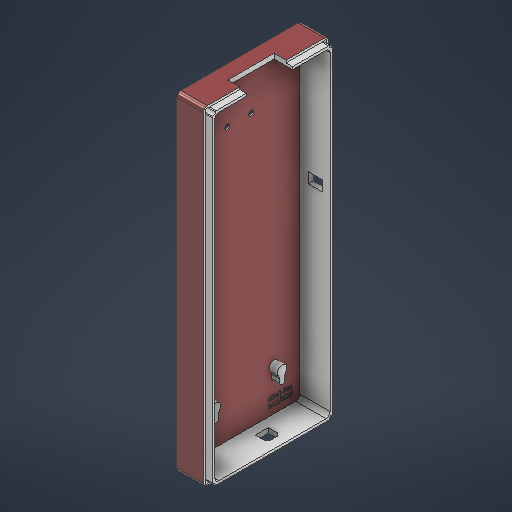
# Autodesk Inventor part: cDAQ_Bottom_Box3
Saved by Autodesk Inventor 2027 (Build 310192000, 192)
## iProperties
Created: 2026-05-08
Part Number: cDAQ_Bottom_Box3
Material: Generic
Document SubType Name: Modeling
Designer: giese
Density: 1 g/cm^3
Appearance: Default
Author: giese
Autodesk Inventor part; units mm, degrees
ref_plane "YZ Plane" through (0, 0, 0) normal (1, 0, 0) x (0, 1, 0)
ref_plane "XZ Plane" through (0, 0, 0) normal (0, 1, 0) x (-1, 0, 0)
ref_plane "XY Plane" through (0, 0, 0) normal (0, 0, 1) x (1, 0, 0)
sketch "Sketch1" plane through (0, 0, 0) normal (1, 0, 0) x (0, 1, 0)
  line L0 (37.5698, 48.0867) -> (-215.7952, 48.0867)
  line L1 (-215.7952, 48.0867) -> (-215.7952, -48.4333)
  line L2 (-215.7952, -48.4333) -> (37.5698, -48.4333)
  line L3 (37.5698, -48.4333) -> (37.5698, 48.0867)
  point P0 (0, 0)
  dimension "d0" = 96.52
  dimension "d1" = 253.365
  constraints: 8 end point, 2 parallel, 1 horizontal, 1 perpendicular
  measures "d0" distance of L2.end L0.start
  measures "d1" distance of L1.end L2.end
extrude "Extrusion1" add sketch "Sketch1" along normal blind 20.32
sketch "Sketch2" plane through (20.32, 0, 0) normal (1, 0, 0) x (0, 0, -1)
  line L0 (44.6233, 33.7598) -> (-44.2767, 33.7598)
  line L1 (-44.2767, 33.7598) -> (-44.2767, -211.9852)
  line L2 (-44.2767, -211.9852) -> (44.6233, -211.9852)
  line L3 (44.6233, -211.9852) -> (44.6233, 33.7598)
  line L4 (48.4333, 37.5698) -> (-48.0867, 37.5698) projected
  line L5 (-48.0867, 37.5698) -> (-48.0867, -215.7952) projected
  point P0 (0, 0)
  dimension "d4" = 245.745
  dimension "d5" = 88.9
  dimension "d8" = 3.81
  dimension "d21" = 3.81
  constraints: 8 end point, 2 parallel, 1 horizontal, 1 perpendicular
  measures "d4" distance of L2.end L0.start
  measures "d5" distance of L0.start L0.end
  measures "d8" distance between parallel lines of L0 L4
  measures "d21" distance between parallel lines of L5 L1
extrude "Extrusion2" cut sketch "Sketch2" against normal blind 18.415
sketch "Sketch3" plane through (0, 0, 0) normal (-1, 0, 0) x (0, 0, 1)
  circle A0 centre (-7.1989, -2.6638) radius 2
  circle A1 centre (11.2999, -2.6638) radius 2
  circle A2 centre (29.7987, -2.6638) radius 2
  line L0 (-48.4333, -215.7952) -> (-48.4333, 37.5698) projected
  line L1 (-48.4333, 37.5698) -> (48.0867, 37.5698) projected
  line L2 (48.0867, 37.5698) -> (48.0867, -215.7952) projected
  line L3 (44.2767, 33.7598) -> (-44.6233, 33.7598) projected
  point P0 (0, 0)
  point P1 (-0.896, -23.7433)
  point P2 (-45.1848, 27.0137)
  dimension "d9" = 18.4988
  dimension "d10" = 4
  dimension "d11" = 4
  dimension "d12" = 18.4988
  dimension "d13" = 36.9976
  dimension "d18" = 18.288
  dimension "d22" = 4
  dimension "d58" = 40.2336
  constraints: 3 centre point
  measures "d9" distance of A0.centre A1.centre
  measures "d10" diameter of A1
  measures "d11" diameter of A2
  measures "d12" distance of A1.centre A2.centre
  measures "d13" distance of A0.centre A2.centre
  measures "d18" distance from line of L2 A2.centre
  measures "d22" diameter of A0
  measures "d58" distance from line of L1 A2.centre
extrude "Extrusion3" cut sketch "Sketch3" against normal blind 3.81
sketch "Sketch5" plane through (0, -215.7952, -48.4333) normal (0, 0, -1) x (-1, 0, 0)
  line L0 (-19.2532, 150.6728) -> (-8.5598, 150.6728)
  line L1 (-8.5598, 150.6728) -> (-8.5598, 158.6728)
  line L2 (-8.5598, 158.6728) -> (-19.2532, 158.6728)
  line L3 (-19.2532, 158.6728) -> (-19.2532, 150.6728)
  line L4 (0, 253.365) -> (-20.32, 253.365) projected
  line L5 (0, 0) -> (0, 253.365) projected
  point P0 (0, 215.7952)
  point P1 (-13.9065, 158.6728)
  point P2 (-13.9065, 150.6728)
  dimension "d28" = 10.6934
  dimension "d30" = 8
  dimension "d31" = 8.5598
  dimension "d34" = 102.6922
  constraints: 8 end point, 2 midpoint, 2 parallel, 1 horizontal, 1 perpendicular
  measures "d28" distance between parallel lines of L1 L3
  measures "d30" distance of point (-13.907, 158.673) point (-13.907, 150.673)
  measures "d31" distance between parallel lines of L5 L1
  measures "d34" distance between parallel lines of L4 L0
extrude "Extrusion4" cut sketch "Sketch5" against normal blind 24.13
sketch "Sketch6" plane through (0, -215.7952, -48.4333) normal (0, -1, 0) x (1, 0, 0)
  line L0 (16, 45.1284) -> (9, 45.1284)
  line L1 (9, 45.1284) -> (9, 35.1284)
  line L2 (9, 35.1284) -> (16, 35.1284)
  line L3 (0, 96.52) -> (0, 0) projected
  line L4 (18.24, 43.1283) -> (18.24, 37.1284)
  line L5 (16, 45.1284) -> (18.24, 43.1283)
  line L6 (18.24, 37.1284) -> (16, 35.1284)
  line L7 (0, 0) -> (20.32, 0) projected
  point P0 (0, 48.4333)
  point P1 (12.5, 45.1284)
  point P2 (12.5, 35.1284)
  dimension "d35" = 10
  dimension "d39" = 6
  dimension "d48" = 45.1284
  dimension "d49" = 18.24
  constraints: 12 end point, 2 midpoint, 1 horizontal, 1 parallel, 1 perpendicular, 1 vertical
  measures "d35" distance of point (12.5, 45.128) point (12.5, 35.128)
  measures "d39" distance of L4.start L4.end
  measures "d48" distance between parallel lines of L7 L0
  measures "d49" distance between parallel lines of L3 L4
extrude "Extrusion5" cut sketch "Sketch6" against normal blind 3.81
sketch "Sketch7" plane through (0, 37.5698, 48.0867) normal (0, 1, 0) x (1, 0, 0)
  line L0 (26.1366, 63.754) -> (11.1252, 63.754)
  line L1 (11.1252, 63.754) -> (11.1252, 28.194)
  line L2 (11.1252, 28.194) -> (26.1366, 28.194)
  line L3 (26.1366, 28.194) -> (26.1366, 63.754)
  line L4 (0, 0) -> (20.32, 0) projected
  line L5 (0, 96.52) -> (0, 0) projected
  line L6 (20.32, 96.52) -> (20.32, 0) projected
  point P0 (0, 48.0867)
  dimension "d51" = 35.56
  dimension "d52" = 28.194
  dimension "d55" = 11.1252
  dimension "d56" = 15.0114
  dimension "d57" = 5.8166
  constraints: 8 end point, 2 parallel, 1 horizontal, 1 perpendicular
  measures "d51" distance of L2.end L0.start
  measures "d52" distance between parallel lines of L4 L2
  measures "d55" distance between parallel lines of L5 L1
  measures "d56" distance between parallel lines of L3 L1
  measures "d57" distance between parallel lines of L6 L3
extrude "Extrusion6" cut sketch "Sketch7" against normal blind 7.62
fillet "Fillet1" radius 3.175 4 edges at (10.16, 37.5698, -48.4333) (10.16, 37.5698, 48.0867) (10.16, -215.7952, -48.4333) (10.16, -215.7952, 48.0867)
sketch "Sketch8" plane through (0, 0, 0) normal (-1, 0, 0) x (0, 0, 1)
  line L0 (-8.9705, -6.1944) -> (-5.4399, -6.1944)
  line L1 (-8.9705, 0.8668) -> (-5.4399, 0.8668)
  line L2 (-8.9705, -6.1944) -> (-11.0089, -2.6638)
  line L3 (-8.9705, 0.8668) -> (-11.0089, -2.6638)
  line L4 (-5.4399, -6.1944) -> (-3.4016, -2.6638)
  line L5 (-5.4399, 0.8668) -> (-3.4016, -2.6638)
  circle A0 centre (-7.1989, -2.6638) radius 2 projected
  line L6 (9.5283, -6.1944) -> (13.0589, -6.1944)
  line L7 (9.5283, 0.8668) -> (13.0589, 0.8668)
  line L8 (9.5283, -6.1944) -> (7.4899, -2.6638)
  line L9 (9.5283, 0.8668) -> (7.4899, -2.6638)
  line L10 (13.0589, -6.1944) -> (15.0973, -2.6638)
  line L11 (13.0589, 0.8668) -> (15.0973, -2.6638)
  circle A1 centre (11.2999, -2.6638) radius 2 projected
  line L12 (28.0271, -6.1944) -> (25.9887, -2.6638)
  line L13 (28.0271, 0.8668) -> (25.9887, -2.6638)
  line L14 (28.0271, -6.1944) -> (31.5577, -6.1944)
  line L15 (28.0271, 0.8668) -> (31.5577, 0.8668)
  line L16 (31.5577, -6.1944) -> (33.5961, -2.6638)
  line L17 (31.5577, 0.8668) -> (33.5961, -2.6638)
  circle A2 centre (29.7987, -2.6638) radius 2 projected
  point P0 (-7.2052, -6.1944)
  point P1 (11.2936, -6.1944)
  point P2 (29.7924, -6.1944)
  point P3 (-11.0089, -2.6638)
  point P4 (-3.4016, -2.6638)
  point P5 (15.0973, -2.6638)
  point P6 (7.4899, -2.6638)
  point P7 (33.5961, -2.6638)
  point P8 (25.9887, -2.6638)
  dimension "d60" = 7.0612
  dimension "d61" = 120
  dimension "d62" = 120
  dimension "d63" = 120
  dimension "d64" = 120
  dimension "d65" = 3.5306
  dimension "d66" = 3.5306
  dimension "d67" = 3.5306
  dimension "d68" = 3.5306
  dimension "d69" = 3.5306
  dimension "d70" = 3.5306
  dimension "d71" = 0
  dimension "d72" = 7.6074
  dimension "d73" = 3.81
  dimension "d74" = 0
  dimension "d75" = 7.0612
  dimension "d76" = 120
  dimension "d77" = 120
  dimension "d78" = 120
  dimension "d79" = 120
  dimension "d80" = 3.5306
  dimension "d81" = 3.5306
  dimension "d82" = 3.5306
  dimension "d83" = 3.5306
  dimension "d84" = 3.5306
  dimension "d85" = 3.5306
  dimension "d86" = 0
  dimension "d87" = 7.6074
  dimension "d91" = 0
  dimension "d92" = 3.81
  dimension "d93" = 7.0612
  dimension "d94" = 120
  dimension "d95" = 120
  dimension "d96" = 120
  dimension "d97" = 120
  dimension "d98" = 3.5306
  dimension "d99" = 3.5306
  dimension "d100" = 3.5306
  dimension "d101" = 3.5306
  dimension "d102" = 3.5306
  dimension "d103" = 3.5306
  dimension "d104" = 0
  dimension "d105" = 7.6074
  dimension "d108" = 0
  dimension "d109" = 3.81
  constraints: 36 end point, 6 horizontal, 3 midpoint
  measures "d60" distance from line of point (-7.205, -6.194) L1
  measures "d61" angle of L0 L2
  measures "d62" angle of L1 L3
  measures "d63" angle of L4 L0
  measures "d64" angle of L5 L1
  measures "d65" distance of L0.start L0.end
  measures "d66" distance of L1.start L1.end
  measures "d67" vertical distance of L1.start L3.end
  measures "d68" vertical distance of L0.start L2.end
  measures "d69" vertical distance of L1.end L5.end
  measures "d70" vertical distance of L0.end L4.end
  measures "d71" horizontal distance of L0.start L1.start
  measures "d72" distance of L4.end L2.end
  measures "d73" distance of A0.centre L2.end
  measures "d74" vertical distance of A0.centre L4.end
  measures "d75" distance from line of point (11.294, -6.194) L7
  measures "d76" angle of L6 L8
  measures "d77" angle of L7 L9
  measures "d78" angle of L10 L6
  measures "d79" angle of L11 L7
  measures "d80" distance of L8.start L6.end
  measures "d81" distance of L9.start L7.end
  measures "d82" vertical distance of L9.start L9.end
  measures "d83" vertical distance of L8.start L8.end
  measures "d84" vertical distance of L7.end L11.end
  measures "d85" vertical distance of L6.end L10.end
  measures "d86" horizontal distance of L8.start L9.start
  measures "d87" distance of L10.end L8.end
  measures "d91" vertical distance of A1.centre L8.end
  measures "d92" distance of A1.centre L8.end
  measures "d93" distance from line of point (29.792, -6.194) L15
  measures "d94" angle of L14 L12
  measures "d95" angle of L15 L13
  measures "d96" angle of L16 L14
  measures "d97" angle of L17 L15
  measures "d98" distance of L12.start L16.start
  measures "d99" distance of L15.start L15.end
  measures "d100" vertical distance of L15.start L13.end
  measures "d101" vertical distance of L12.start L12.end
  measures "d102" vertical distance of L15.end L17.end
  measures "d103" vertical distance of L16.start L16.end
  measures "d104" horizontal distance of L12.start L15.start
  measures "d105" distance of L16.end L12.end
  measures "d108" vertical distance of A2.centre L12.end
  measures "d109" distance of A2.centre L12.end
extrude "Extrusion7" cut sketch "Sketch8" against normal blind 0.9525 contours L2 L3 L1 L5 L4 L0 | A0 | L8 L9 L7 L11 L10 L6 | A1 | L12 L13 L15 L17 L16 L14 | A2
sketch "Sketch9" plane through (1.905, 0, 0) normal (1, 0, 0) x (0, 0, -1)
  arc A0 (27.3489, -182.3284) -> (21.8927, -182.3284) centre (24.6208, -179.8542) ccw
  line L0 (45.2583, 37.5698) -> (15.6673, 37.5698) projected
  line L1 (44.6233, 33.7598) -> (44.6233, -211.9852) projected
  arc A1 (22.7158, -187.4742) -> (26.5258, -187.4742) centre (24.6208, -187.4742) ccw
  line L2 (26.5258, -187.4742) -> (26.5258, -184.4614)
  line L3 (22.7158, -187.4742) -> (22.7158, -184.4614)
  arc A2 (27.3489, -182.3284) -> (26.5258, -184.4614) centre (29.7008, -184.4614) ccw
  arc A3 (22.7158, -184.4614) -> (21.8927, -182.3284) centre (19.5408, -184.4614) ccw
  arc A4 (-23.4511, -182.3284) -> (-28.9073, -182.3285) centre (-26.1792, -179.8542) ccw
  arc A5 (-28.0842, -187.4606) -> (-24.2742, -187.4742) centre (-26.1792, -187.4742) ccw
  line L4 (-24.2742, -187.4742) -> (-24.2742, -184.4614)
  line L5 (-28.0842, -187.4606) -> (-28.0842, -184.4614)
  arc A6 (-23.4511, -182.3284) -> (-24.2742, -184.4614) centre (-21.0992, -184.4614) ccw
  arc A7 (-28.0842, -184.4614) -> (-28.9073, -182.3285) centre (-31.2592, -184.4614) ccw
  line L6 (-19.8927, 37.5698) -> (-44.9117, 37.5698) projected
  line L7 (-44.2767, -211.9852) -> (-44.2767, 33.7598) projected
  point P0 (0, 0)
  point P1 (26.5258, -183.0063)
  point P2 (22.7158, -183.0063)
  point P3 (-24.2742, -183.0063)
  point P4 (-28.0842, -183.0063)
  dimension "d112" = 217.424
  dimension "d114" = 7.366
  dimension "d116" = 3.81
  dimension "d117" = 225.044
  dimension "d118" = 3.175
  dimension "d119" = 7.366
  dimension "d120" = 3.81
  dimension "d121" = 3.175
  dimension "d122" = 217.424
  dimension "d123" = 225.044
  dimension "d125" = 0
  dimension "d128" = 50.8
  dimension "d129" = 20.0025
  dimension "d130" = 0
  constraints: 20 point on circle, 8 centre point, 8 end point, 8 tangent, 4 point on line, 2 equal radius, 2 parallel, 2 vertical
  measures "d112" distance from line of L0 A0.centre
  measures "d114" diameter of A0
  measures "d116" diameter of A1
  measures "d117" distance from line of L0 A1.centre
  measures "d118" radius of A2
  measures "d119" diameter of A4
  measures "d120" diameter of A5
  measures "d121" radius of A6
  measures "d122" distance from line of A4.centre L6
  measures "d123" distance from line of L6 A5.centre
  measures "d125" horizontal distance of A5.centre A4.centre
  measures "d128" distance of A5.centre A1.centre
  measures "d129" distance from line of L1 A0.centre
  measures "d130" horizontal distance of A0.centre A1.centre
extrude "Extrusion8" add sketch "Sketch9" along normal blind 6.4008
sketch "Sketch10" plane through (20.32, 0, 0) normal (1, 0, 0) x (0, 0, -1)
  line L0 (44.6233, -211.9852) -> (-44.2767, -211.9852) projected
  line L1 (-44.2767, -211.9852) -> (-44.2767, 33.7598) projected
  line L2 (-44.2767, -211.9852) -> (-44.2767, -209.6992)
  line L3 (-46.2767, -211.4452) -> (-46.2767, -213.9852)
  line L4 (-46.2767, -213.9852) -> (-41.9907, -213.9852)
  line L5 (-44.2767, -211.9852) -> (-41.9907, -211.9852)
  line L6 (44.6233, -211.9852) -> (42.3373, -211.9852)
  line L7 (42.3373, -213.9852) -> (46.6233, -213.9852)
  line L8 (46.6233, -213.9852) -> (46.6233, -209.6992)
  line L9 (44.6233, 33.7598) -> (44.6233, -211.9852) projected
  line L10 (-44.2767, -209.6992) -> (-44.2767, 33.7598)
  line L11 (-44.2767, 33.7598) -> (44.6233, 33.7598) projected
  line L12 (-41.9907, 35.7598) -> (-46.2767, 35.7598)
  line L13 (-46.2767, 35.7598) -> (-46.2767, 29.7278)
  line L14 (42.3373, 33.7598) -> (44.6233, 33.7598)
  line L15 (46.6233, 31.4738) -> (46.6233, 35.7598)
  line L16 (46.6233, 35.7598) -> (42.3373, 35.7598)
  line L17 (-41.9907, -213.9852) -> (42.3373, -213.9852)
  line L18 (42.3373, -211.9852) -> (-41.9907, -211.9852)
  line L19 (46.6233, -209.6992) -> (46.6233, 31.4738)
  line L20 (44.6233, 31.4738) -> (44.6233, -209.6992)
  line L21 (42.3373, 33.7598) -> (-41.9907, 33.7598)
  line L22 (-41.9907, 35.7598) -> (42.3373, 35.7598)
  line L23 (-44.2767, -209.6992) -> (-44.2767, -209.6992)
  line L24 (-46.2767, 29.7278) -> (-46.2767, -211.4452)
  point P0 (-41.9907, -213.8582)
  point P1 (-44.4037, -209.6992)
  point P2 (-46.2767, 32.7438)
  point P3 (44.6233, 31.4738)
  point P4 (42.3373, 35.7598)
  dimension "d139" = 2
  dimension "d142" = 2
  dimension "d143" = 2
  dimension "d146" = 2
  dimension "d147" = 2
  dimension "d150" = 2
  dimension "d151" = 2
  dimension "d159" = 2
  constraints: 42 end point, 7 point on line, 4 perpendicular, 3 horizontal, 3 parallel, 2 vertical, 1 collinear, 1 midpoint
  measures "d139" distance between parallel lines of L0 L4
  measures "d142" distance between parallel lines of L6 L7
  measures "d143" distance between parallel lines of L9 L8
  measures "d146" distance from line of point (-46.277, 32.744) L1
  measures "d147" distance between parallel lines of L11 L12
  measures "d150" distance between parallel lines of L11 L16
  measures "d151" distance between parallel lines of L9 L15
  measures "d159" distance from line of L1 L3.start
extrude "Extrusion9" add sketch "Sketch10" along normal blind 5
sketch "Sketch11" plane through (20.32, 35.7598, 19.8927) normal (0, 1, 0) x (1, 0, 0)
  line L0 (0, 35.56) -> (-9.1948, 35.56) projected
  line L1 (5, 66.516) -> (5, -26.384) projected
  line L2 (0, 35.56) -> (5, 35.56)
  line L3 (5, 35.56) -> (5, 0)
  line L4 (5, 0) -> (0, 0)
  line L5 (0, 0) -> (0, 35.56)
  point P0 (-20.32, 19.8927)
  point P1 (2.5, 0)
  point P2 (2.5, 35.56)
  point P3 (5, 35.56)
  dimension "d156" = 35.56
  constraints: 8 end point, 2 midpoint, 2 parallel, 1 horizontal, 1 perpendicular, 1 point on line
  measures "d156" distance of point (2.5, 0) point (2.5, 35.56)
extrude "Extrusion10" cut sketch "Sketch11" against normal blind 9.8425
fillet "Fillet2" radius 3.175 8 edges at (22.82, 35.7598, -46.6233) (22.82, 35.7598, 46.2767) (22.82, -213.9852, 46.2767) (22.82, -213.9852, -46.6233) (13.6125, 33.7598, -44.6233) (13.6125, 33.7598, 44.2767) (13.6125, -211.9852, 44.2767) (13.6125, -211.9852, -44.6233)
sketch "Sketch13" plane through (25.32, 0, 0) normal (1, 0, 0) x (0, 0, -1)
  arc A0 (46.6233, 32.5848) -> (43.4483, 35.7598) centre (43.4483, 32.5848) ccw projected
  arc A1 (-43.1017, 35.7598) -> (-46.2767, 32.5848) centre (-43.1017, 32.5848) ccw projected
  circle A2 centre (-45.3344, 34.8421) radius 1.5
  arc A3 (43.4483, -213.9852) -> (46.6233, -210.8102) centre (43.4483, -210.8102) ccw projected
  circle A4 centre (45.681, -213.0676) radius 1.5
  arc A5 (-46.2767, -210.8102) -> (-43.1017, -213.9852) centre (-43.1017, -210.8102) ccw projected
  circle A6 centre (-45.3344, -213.0676) radius 1.5
  circle A7 centre (45.681, 34.8421) radius 1.5
  line L0 (-19.8927, 37.5698) -> (-44.9117, 37.5698) projected
  line L1 (-48.0867, 34.3948) -> (-48.0867, -212.6202) projected
  point P0 (0, 0)
  point P1 (-45.3468, 34.8298)
  dimension "d166" = 3
  dimension "d167" = 3
  dimension "d168" = 3
  dimension "d169" = 3
  dimension "d170" = 2.7399
  dimension "d171" = 2.7523
  constraints: 5 point on circle, 4 centre point
  measures "d166" diameter of A6
  measures "d167" diameter of A4
  measures "d168" diameter of A2
  measures "d169" diameter of A7
  measures "d170" distance from line of L0 point (-45.347, 34.83)
  measures "d171" distance from line of L1 A2.centre
extrude "Extrusion11" cut sketch "Sketch13" against normal blind 25.4
sketch "Sketch14" plane through (1.905, 0, 0) normal (1, 0, 0) x (0, 0, -1)
  line L0 (20.2548, -198.8409) -> (39.4715, -198.8409) construction
  line L1 (39.4715, -198.8409) -> (39.4715, -207.6335) construction
  line L2 (39.4715, -207.6335) -> (20.2548, -207.6335) construction
  line L3 (20.2548, -207.6335) -> (20.2548, -198.8409) construction
  spline S0 degree 2 poles (21.4428, -202.005) (21.2057, -202.005) (20.813, -201.8592) (20.6722, -201.711) knots 0 0 0 1 2 2 2
  spline S1 degree 2 poles (20.6722, -201.711) (20.5314, -201.5653) (20.3758, -201.1158) (20.3758, -200.8144) knots 0 0 0 1 2 2 2
  spline S2 degree 2 poles (20.3758, -200.8144) (20.3758, -200.5131) (20.5363, -200.0734) (20.6722, -199.9252) knots 0 0 0 1 2 2 2
  spline S3 degree 2 poles (20.6722, -199.9252) (20.808, -199.7745) (21.2107, -199.614) (21.4428, -199.614) knots 0 0 0 1 2 2 2
  spline S4 degree 2 poles (21.4428, -199.614) (21.6306, -199.614) (21.9813, -199.7202) (22.1172, -199.7894) knots 0 0 0 1 2 2 2
  line L4 (22.1172, -199.7894) -> (22.1172, -200.2216)
  line L5 (22.1172, -200.2216) -> (22.0949, -200.2216)
  spline S5 degree 2 poles (22.0949, -200.2216) (22.0529, -200.187) (21.9245, -200.0981) (21.8331, -200.0512) knots 0 0 0 1 2 2 2
  spline S6 degree 2 poles (21.8331, -200.0512) (21.7516, -200.0117) (21.5342, -199.9499) (21.4354, -199.9499) knots 0 0 0 1 2 2 2
  spline S7 degree 2 poles (21.4354, -199.9499) (21.1366, -199.9499) (20.7735, -200.4019) (20.7735, -200.8144) knots 0 0 0 1 2 2 2
  spline S8 degree 2 poles (20.7735, -200.8144) (20.7735, -201.217) (21.1242, -201.669) (21.4354, -201.669) knots 0 0 0 1 2 2 2
  spline S9 degree 2 poles (21.4354, -201.669) (21.6231, -201.669) (21.964, -201.5134) (22.0949, -201.3924) knots 0 0 0 1 2 2 2
  line L6 (22.0949, -201.3924) -> (22.1172, -201.3924)
  line L7 (22.1172, -201.3924) -> (22.1172, -201.8247)
  spline S10 degree 2 poles (22.1172, -201.8247) (22.0603, -201.8518) (21.8874, -201.9284) (21.8183, -201.9457) knots 0 0 0 1 2 2 2
  spline S11 degree 2 poles (21.8183, -201.9457) (21.7195, -201.9753) (21.5639, -202.005) (21.4428, -202.005) knots 0 0 0 1 2 2 2
  spline S12 degree 2 poles (24.9009, -200.4316) (24.9009, -200.849) (24.5625, -201.5208) (24.2784, -201.7086) knots 0 0 0 1 2 2 2
  spline S13 degree 2 poles (24.2784, -201.7086) (24.0462, -201.8543) (23.5695, -201.9531) (23.199, -201.9531) knots 0 0 0 1 2 2 2
  line L8 (23.199, -201.9531) -> (22.4975, -201.9531)
  line L9 (22.4975, -201.9531) -> (22.4975, -198.9051)
  line L10 (22.4975, -198.9051) -> (23.1916, -198.9051)
  spline S14 degree 2 poles (23.1916, -198.9051) (23.6214, -198.9051) (24.1105, -199.0335) (24.2834, -199.1472) knots 0 0 0 1 2 2 2
  spline S15 degree 2 poles (24.2834, -199.1472) (24.5773, -199.3423) (24.9009, -199.987) (24.9009, -200.4316) knots 0 0 0 1 2 2 2
  spline S16 degree 2 poles (24.4785, -200.4266) (24.4785, -200.0759) (24.2463, -199.5794) (24.0166, -199.4386) knots 0 0 0 1 2 2 2
  spline S17 degree 2 poles (24.0166, -199.4386) (23.8536, -199.3423) (23.4855, -199.2558) (23.2114, -199.2558) knots 0 0 0 1 2 2 2
  line L11 (23.2114, -199.2558) -> (22.9026, -199.2558)
  line L12 (22.9026, -199.2558) -> (22.9026, -201.6024)
  line L13 (22.9026, -201.6024) -> (23.2114, -201.6024)
  spline S18 degree 2 poles (23.2114, -201.6024) (23.4806, -201.6024) (23.8882, -201.5159) (24.0536, -201.3998) knots 0 0 0 1 2 2 2
  spline S19 degree 2 poles (24.0536, -201.3998) (24.2661, -201.2566) (24.4785, -200.7823) (24.4785, -200.4266) knots 0 0 0 1 2 2 2
  line L14 (25.012, -201.9531) -> (26.0395, -198.9051)
  line L15 (26.0395, -198.9051) -> (26.5385, -198.9051)
  line L16 (26.5385, -198.9051) -> (27.566, -201.9531)
  line L17 (27.566, -201.9531) -> (27.1387, -201.9531)
  line L18 (27.1387, -201.9531) -> (26.8621, -201.1009)
  line L19 (26.8621, -201.1009) -> (25.6987, -201.1009)
  line L20 (25.6987, -201.1009) -> (25.422, -201.9531)
  line L21 (25.422, -201.9531) -> (25.012, -201.9531)
  line L22 (26.7509, -200.7551) -> (26.2791, -199.3201)
  line L23 (26.2791, -199.3201) -> (25.8098, -200.7551)
  line L24 (25.8098, -200.7551) -> (26.7509, -200.7551)
  spline S20 degree 2 poles (30.3868, -202.699) (30.2756, -202.7262) (30.0336, -202.7559) (29.9125, -202.7559) knots 0 0 0 1 2 2 2
  spline S21 degree 2 poles (29.9125, -202.7559) (29.5692, -202.7559) (29.1419, -202.373) (29.1221, -202.0173) knots 0 0 0 1 2 2 2
  spline S22 degree 2 poles (29.1221, -202.0173) (29.0949, -202.0173) (29.048, -202.0173) (29.0283, -202.0173) knots 0 0 0 1 2 2 2
  spline S23 degree 2 poles (29.0283, -202.0173) (28.7195, -202.0173) (28.223, -201.8074) (28.0452, -201.6024) knots 0 0 0 1 2 2 2
  spline S24 degree 2 poles (28.0452, -201.6024) (27.8698, -201.3998) (27.6821, -200.807) (27.6821, -200.4316) knots 0 0 0 1 2 2 2
  spline S25 degree 2 poles (27.6821, -200.4316) (27.6821, -200.0462) (27.8723, -199.4633) (28.0477, -199.2558) knots 0 0 0 1 2 2 2
  spline S26 degree 2 poles (28.0477, -199.2558) (28.2255, -199.0508) (28.722, -198.8409) (29.0283, -198.8409) knots 0 0 0 1 2 2 2
  spline S27 degree 2 poles (29.0283, -198.8409) (29.3395, -198.8409) (29.8384, -199.0582) (30.0113, -199.2558) knots 0 0 0 1 2 2 2
  spline S28 degree 2 poles (30.0113, -199.2558) (30.1842, -199.4559) (30.3769, -200.0512) (30.3769, -200.4316) knots 0 0 0 1 2 2 2
  spline S29 degree 2 poles (30.3769, -200.4316) (30.3769, -201.0244) (29.915, -201.795) (29.5124, -201.9309) knots 0 0 0 1 2 2 2
  spline S30 degree 2 poles (29.5124, -201.9309) (29.5223, -202.0445) (29.5815, -202.2273) (29.6285, -202.2791) knots 0 0 0 1 2 2 2
  spline S31 degree 2 poles (29.6285, -202.2791) (29.6853, -202.3434) (29.8409, -202.4026) (29.9792, -202.4026) knots 0 0 0 1 2 2 2
  spline S32 degree 2 poles (29.9792, -202.4026) (30.0607, -202.4026) (30.283, -202.3508) (30.3324, -202.331) knots 0 0 0 1 2 2 2
  line L25 (30.3324, -202.331) -> (30.3868, -202.331)
  line L26 (30.3868, -202.331) -> (30.3868, -202.699)
  spline S33 degree 2 poles (29.9545, -200.4316) (29.9545, -200.1278) (29.8236, -199.6609) (29.705, -199.5078) knots 0 0 0 1 2 2 2
  spline S34 degree 2 poles (29.705, -199.5078) (29.584, -199.3497) (29.2431, -199.1916) (29.0307, -199.1916) knots 0 0 0 1 2 2 2
  spline S35 degree 2 poles (29.0307, -199.1916) (28.8109, -199.1916) (28.4799, -199.3448) (28.3539, -199.5078) knots 0 0 0 1 2 2 2
  spline S36 degree 2 poles (28.3539, -199.5078) (28.2329, -199.6634) (28.1045, -200.1352) (28.1045, -200.4316) knots 0 0 0 1 2 2 2
  spline S37 degree 2 poles (28.1045, -200.4316) (28.1045, -201.0318) (28.6084, -201.6715) (29.0307, -201.6715) knots 0 0 0 1 2 2 2
  spline S38 degree 2 poles (29.0307, -201.6715) (29.4531, -201.6715) (29.9545, -201.0318) (29.9545, -200.4316) knots 0 0 0 1 2 2 2
  spline S39 degree 2 poles (34.198, -201.017) (34.198, -201.2442) (34.0251, -201.5925) (33.8818, -201.7061) knots 0 0 0 1 2 2 2
  spline S40 degree 2 poles (33.8818, -201.7061) (33.7089, -201.8395) (33.3162, -201.9531) (33.005, -201.9531) knots 0 0 0 1 2 2 2
  line L27 (33.005, -201.9531) -> (32.1306, -201.9531)
  line L28 (32.1306, -201.9531) -> (32.1306, -198.9051)
  line L29 (32.1306, -198.9051) -> (32.9383, -198.9051)
  spline S41 degree 2 poles (32.9383, -198.9051) (33.2643, -198.9051) (33.5904, -198.9471) (33.7386, -199.0286) knots 0 0 0 1 2 2 2
  spline S42 degree 2 poles (33.7386, -199.0286) (33.9041, -199.1151) (34.0547, -199.3991) (34.0547, -199.5918) knots 0 0 0 1 2 2 2
  spline S43 degree 2 poles (34.0547, -199.5918) (34.0547, -199.8067) (33.8275, -200.1475) (33.6274, -200.2438) knots 0 0 0 1 2 2 2
  line L30 (33.6274, -200.2438) -> (33.6274, -200.2587)
  spline S44 degree 2 poles (33.6274, -200.2587) (33.8991, -200.3328) (34.198, -200.7255) (34.198, -201.017) knots 0 0 0 1 2 2 2
  spline S45 degree 2 poles (33.7756, -201.0343) (33.7756, -200.8614) (33.6768, -200.6391) (33.5286, -200.56) knots 0 0 0 1 2 2 2
  spline S46 degree 2 poles (33.5286, -200.56) (33.4323, -200.5106) (33.2051, -200.481) (32.9951, -200.481) knots 0 0 0 1 2 2 2
  line L31 (32.9951, -200.481) -> (32.5357, -200.481)
  line L32 (32.5357, -200.481) -> (32.5357, -201.6073)
  line L33 (32.5357, -201.6073) -> (32.8642, -201.6073)
  spline S47 degree 2 poles (32.8642, -201.6073) (33.131, -201.6073) (33.4372, -201.5579) (33.5558, -201.4789) knots 0 0 0 1 2 2 2
  spline S48 degree 2 poles (33.5558, -201.4789) (33.6694, -201.3973) (33.7756, -201.1948) (33.7756, -201.0343) knots 0 0 0 1 2 2 2
  spline S49 degree 2 poles (33.6324, -199.6486) (33.6324, -199.5399) (33.5583, -199.3769) (33.4768, -199.3299) knots 0 0 0 1 2 2 2
  spline S50 degree 2 poles (33.4768, -199.3299) (33.378, -199.2756) (33.1384, -199.2509) (32.9235, -199.2509) knots 0 0 0 1 2 2 2
  line L34 (32.9235, -199.2509) -> (32.5357, -199.2509)
  line L35 (32.5357, -199.2509) -> (32.5357, -200.1426)
  line L36 (32.5357, -200.1426) -> (32.9951, -200.1426)
  spline S51 degree 2 poles (32.9951, -200.1426) (33.1853, -200.1426) (33.3656, -200.1031) (33.4619, -200.0413) knots 0 0 0 1 2 2 2
  spline S52 degree 2 poles (33.4619, -200.0413) (33.5558, -199.982) (33.6324, -199.7918) (33.6324, -199.6486) knots 0 0 0 1 2 2 2
  spline S53 degree 2 poles (36.4507, -200.8095) (36.4507, -201.3875) (35.8949, -202.0173) (35.4305, -202.0173) knots 0 0 0 1 2 2 2
  spline S54 degree 2 poles (35.4305, -202.0173) (34.9538, -202.0173) (34.408, -201.3677) (34.408, -200.8095) knots 0 0 0 1 2 2 2
  spline S55 degree 2 poles (34.408, -200.8095) (34.408, -200.2364) (34.9711, -199.6016) (35.4305, -199.6016) knots 0 0 0 1 2 2 2
  spline S56 degree 2 poles (35.4305, -199.6016) (35.8949, -199.6016) (36.4507, -200.234) (36.4507, -200.8095) knots 0 0 0 1 2 2 2
  spline S57 degree 2 poles (36.053, -200.8095) (36.053, -200.3649) (35.7294, -199.9326) (35.4305, -199.9326) knots 0 0 0 1 2 2 2
  spline S58 degree 2 poles (35.4305, -199.9326) (35.1317, -199.9326) (34.8056, -200.3649) (34.8056, -200.8095) knots 0 0 0 1 2 2 2
  spline S59 degree 2 poles (34.8056, -200.8095) (34.8056, -201.2417) (35.1317, -201.6863) (35.4305, -201.6863) knots 0 0 0 1 2 2 2
  spline S60 degree 2 poles (35.4305, -201.6863) (35.7269, -201.6863) (36.053, -201.2491) (36.053, -200.8095) knots 0 0 0 1 2 2 2
  line L37 (38.6218, -201.9531) -> (38.15, -201.9531)
  line L38 (38.15, -201.9531) -> (37.5943, -201.0935)
  line L39 (37.5943, -201.0935) -> (37.0237, -201.9531)
  line L40 (37.0237, -201.9531) -> (36.5865, -201.9531)
  line L41 (36.5865, -201.9531) -> (37.3794, -200.8194)
  line L42 (37.3794, -200.8194) -> (36.5939, -199.6659)
  line L43 (36.5939, -199.6659) -> (37.0657, -199.6659)
  line L44 (37.0657, -199.6659) -> (37.619, -200.518)
  line L45 (37.619, -200.518) -> (38.1846, -199.6659)
  line L46 (38.1846, -199.6659) -> (38.6218, -199.6659)
  line L47 (38.6218, -199.6659) -> (37.8339, -200.7947)
  line L48 (37.8339, -200.7947) -> (38.6218, -201.9531)
  spline S61 degree 2 poles (22.3246, -206.0033) (22.3246, -206.2231) (22.1838, -206.5986) (22.0554, -206.7369) knots 0 0 0 1 2 2 2
  spline S62 degree 2 poles (22.0554, -206.7369) (21.927, -206.8752) (21.5441, -207.0358) (21.307, -207.0358) knots 0 0 0 1 2 2 2
  spline S63 degree 2 poles (21.307, -207.0358) (21.0896, -207.0358) (20.6648, -206.9394) (20.5092, -206.8629) knots 0 0 0 1 2 2 2
  line L49 (20.5092, -206.8629) -> (20.5092, -206.4306)
  line L50 (20.5092, -206.4306) -> (20.5388, -206.4306)
  spline S64 degree 2 poles (20.5388, -206.4306) (20.5857, -206.4652) (20.7611, -206.5541) (20.8673, -206.5936) knots 0 0 0 1 2 2 2
  spline S65 degree 2 poles (20.8673, -206.5936) (20.9884, -206.6356) (21.1884, -206.6826) (21.3144, -206.6826) knots 0 0 0 1 2 2 2
  spline S66 degree 2 poles (21.3144, -206.6826) (21.4379, -206.6826) (21.6701, -206.5936) (21.7541, -206.4973) knots 0 0 0 1 2 2 2
  spline S67 degree 2 poles (21.7541, -206.4973) (21.8306, -206.4059) (21.9097, -206.1639) (21.9097, -206.0008) knots 0 0 0 1 2 2 2
  spline S68 degree 2 poles (21.9097, -206.0008) (21.9097, -205.8378) (21.8207, -205.6303) (21.7368, -205.5612) knots 0 0 0 1 2 2 2
  spline S69 degree 2 poles (21.7368, -205.5612) (21.6503, -205.4846) (21.3934, -205.4204) (21.2378, -205.4204) knots 0 0 0 1 2 2 2
  spline S70 degree 2 poles (21.2378, -205.4204) (21.0699, -205.4204) (20.7364, -205.4723) (20.6351, -205.4945) knots 0 0 0 1 2 2 2
  line L51 (20.6351, -205.4945) -> (20.6351, -203.9236)
  line L52 (20.6351, -203.9236) -> (22.3073, -203.9236)
  line L53 (22.3073, -203.9236) -> (22.3073, -204.2817)
  line L54 (22.3073, -204.2817) -> (21.0279, -204.2817)
  line L55 (21.0279, -204.2817) -> (21.0279, -205.0943)
  spline S71 degree 2 poles (21.0279, -205.0943) (21.102, -205.0845) (21.2452, -205.0771) (21.3045, -205.0771) knots 0 0 0 1 2 2 2
  spline S72 degree 2 poles (21.3045, -205.0771) (21.5392, -205.0771) (21.8627, -205.1536) (22.0109, -205.2672) knots 0 0 0 1 2 2 2
  spline S73 degree 2 poles (22.0109, -205.2672) (22.1616, -205.3809) (22.3246, -205.7267) (22.3246, -206.0033) knots 0 0 0 1 2 2 2
  line L56 (24.0314, -203.7877) -> (22.8384, -207.6335)
  line L57 (22.8384, -207.6335) -> (22.4926, -207.6335)
  line L58 (22.4926, -207.6335) -> (23.6807, -203.7877)
  line L59 (23.6807, -203.7877) -> (24.0314, -203.7877)
  line L60 (26.247, -206.9716) -> (24.3673, -206.9716)
  line L61 (24.3673, -206.9716) -> (24.3673, -206.5393)
  spline S74 degree 2 poles (24.3673, -206.5393) (24.5699, -206.3491) (24.9305, -205.9959) (25.1034, -205.8057) knots 0 0 0 1 2 2 2
  spline S75 degree 2 poles (25.1034, -205.8057) (25.4517, -205.4229) (25.7061, -204.9634) (25.7061, -204.7189) knots 0 0 0 1 2 2 2
  spline S76 degree 2 poles (25.7061, -204.7189) (25.7061, -204.5905) (25.627, -204.3978) (25.5554, -204.336) knots 0 0 0 1 2 2 2
  spline S77 degree 2 poles (25.5554, -204.336) (25.4838, -204.2743) (25.2961, -204.2125) (25.1824, -204.2125) knots 0 0 0 1 2 2 2
  spline S78 degree 2 poles (25.1824, -204.2125) (25.0738, -204.2125) (24.8515, -204.2669) (24.7502, -204.3089) knots 0 0 0 1 2 2 2
  spline S79 degree 2 poles (24.7502, -204.3089) (24.6637, -204.3435) (24.5032, -204.4423) (24.4538, -204.4768) knots 0 0 0 1 2 2 2
  line L62 (24.4538, -204.4768) -> (24.4316, -204.4768)
  line L63 (24.4316, -204.4768) -> (24.4316, -204.0421)
  spline S80 degree 2 poles (24.4316, -204.0421) (24.5575, -203.9804) (25.0095, -203.8593) (25.2121, -203.8593) knots 0 0 0 1 2 2 2
  spline S81 degree 2 poles (25.2121, -203.8593) (25.6394, -203.8593) (26.121, -204.3113) (26.121, -204.6967) knots 0 0 0 1 2 2 2
  spline S82 degree 2 poles (26.121, -204.6967) (26.121, -204.877) (26.0371, -205.1783) (25.963, -205.3068) knots 0 0 0 1 2 2 2
  spline S83 degree 2 poles (25.963, -205.3068) (25.8889, -205.4401) (25.674, -205.702) (25.5554, -205.8279) knots 0 0 0 1 2 2 2
  spline S84 degree 2 poles (25.5554, -205.8279) (25.3628, -206.0379) (24.891, -206.4874) (24.7502, -206.6183) knots 0 0 0 1 2 2 2
  line L64 (24.7502, -206.6183) -> (26.247, -206.6183)
  line L65 (26.247, -206.6183) -> (26.247, -206.9716)
  line L66 (28.3811, -206.9716) -> (26.8942, -206.9716)
  line L67 (26.8942, -206.9716) -> (26.8942, -206.6603)
  line L68 (26.8942, -206.6603) -> (27.4474, -206.6603)
  line L69 (27.4474, -206.6603) -> (27.4474, -204.6176)
  line L70 (27.4474, -204.6176) -> (26.8942, -204.6176)
  line L71 (26.8942, -204.6176) -> (26.8942, -204.3385)
  spline S85 degree 2 poles (26.8942, -204.3385) (27.2079, -204.3385) (27.5043, -204.1607) (27.524, -203.9137) knots 0 0 0 1 2 2 2
  line L72 (27.524, -203.9137) -> (27.8402, -203.9137)
  line L73 (27.8402, -203.9137) -> (27.8402, -206.6603)
  line L74 (27.8402, -206.6603) -> (28.3811, -206.6603)
  line L75 (28.3811, -206.6603) -> (28.3811, -206.9716)
  line L76 (30.2089, -203.7877) -> (29.0159, -207.6335)
  line L77 (29.0159, -207.6335) -> (28.6701, -207.6335)
  line L78 (28.6701, -207.6335) -> (29.8582, -203.7877)
  line L79 (29.8582, -203.7877) -> (30.2089, -203.7877)
  line L80 (32.4245, -206.9716) -> (30.5448, -206.9716)
  line L81 (30.5448, -206.9716) -> (30.5448, -206.5393)
  spline S86 degree 2 poles (30.5448, -206.5393) (30.7474, -206.3491) (31.108, -205.9959) (31.2809, -205.8057) knots 0 0 0 1 2 2 2
  spline S87 degree 2 poles (31.2809, -205.8057) (31.6292, -205.4229) (31.8836, -204.9634) (31.8836, -204.7189) knots 0 0 0 1 2 2 2
  spline S88 degree 2 poles (31.8836, -204.7189) (31.8836, -204.5905) (31.8046, -204.3978) (31.7329, -204.336) knots 0 0 0 1 2 2 2
  spline S89 degree 2 poles (31.7329, -204.336) (31.6613, -204.2743) (31.4736, -204.2125) (31.36, -204.2125) knots 0 0 0 1 2 2 2
  spline S90 degree 2 poles (31.36, -204.2125) (31.2513, -204.2125) (31.029, -204.2669) (30.9277, -204.3089) knots 0 0 0 1 2 2 2
  spline S91 degree 2 poles (30.9277, -204.3089) (30.8412, -204.3435) (30.6807, -204.4423) (30.6313, -204.4768) knots 0 0 0 1 2 2 2
  line L82 (30.6313, -204.4768) -> (30.6091, -204.4768)
  line L83 (30.6091, -204.4768) -> (30.6091, -204.0421)
  spline S92 degree 2 poles (30.6091, -204.0421) (30.735, -203.9804) (31.187, -203.8593) (31.3896, -203.8593) knots 0 0 0 1 2 2 2
  spline S93 degree 2 poles (31.3896, -203.8593) (31.8169, -203.8593) (32.2986, -204.3113) (32.2986, -204.6967) knots 0 0 0 1 2 2 2
  spline S94 degree 2 poles (32.2986, -204.6967) (32.2986, -204.877) (32.2146, -205.1783) (32.1405, -205.3068) knots 0 0 0 1 2 2 2
  spline S95 degree 2 poles (32.1405, -205.3068) (32.0664, -205.4401) (31.8515, -205.702) (31.7329, -205.8279) knots 0 0 0 1 2 2 2
  spline S96 degree 2 poles (31.7329, -205.8279) (31.5403, -206.0379) (31.0685, -206.4874) (30.9277, -206.6183) knots 0 0 0 1 2 2 2
  line L84 (30.9277, -206.6183) -> (32.4245, -206.6183)
  line L85 (32.4245, -206.6183) -> (32.4245, -206.9716)
  spline S97 degree 2 poles (34.7291, -205.4476) (34.7291, -206.2676) (34.2523, -207.0358) (33.7559, -207.0358) knots 0 0 0 1 2 2 2
  spline S98 degree 2 poles (33.7559, -207.0358) (33.252, -207.0358) (32.7802, -206.2528) (32.7802, -205.45) knots 0 0 0 1 2 2 2
  spline S99 degree 2 poles (32.7802, -205.45) (32.7802, -204.625) (33.2569, -203.8618) (33.7559, -203.8618) knots 0 0 0 1 2 2 2
  spline S100 degree 2 poles (33.7559, -203.8618) (34.2573, -203.8618) (34.7291, -204.6522) (34.7291, -205.4476) knots 0 0 0 1 2 2 2
  spline S101 degree 2 poles (34.2054, -206.3763) (34.2647, -206.2256) (34.3141, -205.7612) (34.3141, -205.4476) knots 0 0 0 1 2 2 2
  spline S102 degree 2 poles (34.3141, -205.4476) (34.3141, -205.1339) (34.2647, -204.672) (34.2029, -204.5164) knots 0 0 0 1 2 2 2
  spline S103 degree 2 poles (34.2029, -204.5164) (34.1412, -204.3607) (33.9263, -204.2002) (33.7559, -204.2002) knots 0 0 0 1 2 2 2
  spline S104 degree 2 poles (33.7559, -204.2002) (33.5854, -204.2002) (33.3656, -204.3607) (33.3014, -204.5213) knots 0 0 0 1 2 2 2
  spline S105 degree 2 poles (33.3014, -204.5213) (33.2396, -204.6769) (33.1952, -205.1512) (33.1952, -205.45) knots 0 0 0 1 2 2 2
  spline S106 degree 2 poles (33.1952, -205.45) (33.1952, -205.7711) (33.2347, -206.2009) (33.2989, -206.3689) knots 0 0 0 1 2 2 2
  spline S107 degree 2 poles (33.2989, -206.3689) (33.3582, -206.527) (33.578, -206.6974) (33.7559, -206.6974) knots 0 0 0 1 2 2 2
  spline S108 degree 2 poles (33.7559, -206.6974) (33.9238, -206.6974) (34.1437, -206.5368) (34.2054, -206.3763) knots 0 0 0 1 2 2 2
  line L86 (36.999, -206.9716) -> (35.1193, -206.9716)
  line L87 (35.1193, -206.9716) -> (35.1193, -206.5393)
  spline S109 degree 2 poles (35.1193, -206.5393) (35.3219, -206.3491) (35.6825, -205.9959) (35.8554, -205.8057) knots 0 0 0 1 2 2 2
  spline S110 degree 2 poles (35.8554, -205.8057) (36.2037, -205.4229) (36.4581, -204.9634) (36.4581, -204.7189) knots 0 0 0 1 2 2 2
  spline S111 degree 2 poles (36.4581, -204.7189) (36.4581, -204.5905) (36.379, -204.3978) (36.3074, -204.336) knots 0 0 0 1 2 2 2
  spline S112 degree 2 poles (36.3074, -204.336) (36.2358, -204.2743) (36.048, -204.2125) (35.9344, -204.2125) knots 0 0 0 1 2 2 2
  spline S113 degree 2 poles (35.9344, -204.2125) (35.8257, -204.2125) (35.6034, -204.2669) (35.5022, -204.3089) knots 0 0 0 1 2 2 2
  spline S114 degree 2 poles (35.5022, -204.3089) (35.4157, -204.3435) (35.2552, -204.4423) (35.2058, -204.4768) knots 0 0 0 1 2 2 2
  line L88 (35.2058, -204.4768) -> (35.1835, -204.4768)
  line L89 (35.1835, -204.4768) -> (35.1835, -204.0421)
  spline S115 degree 2 poles (35.1835, -204.0421) (35.3095, -203.9804) (35.7615, -203.8593) (35.9641, -203.8593) knots 0 0 0 1 2 2 2
  spline S116 degree 2 poles (35.9641, -203.8593) (36.3914, -203.8593) (36.873, -204.3113) (36.873, -204.6967) knots 0 0 0 1 2 2 2
  spline S117 degree 2 poles (36.873, -204.6967) (36.873, -204.877) (36.789, -205.1783) (36.7149, -205.3068) knots 0 0 0 1 2 2 2
  spline S118 degree 2 poles (36.7149, -205.3068) (36.6408, -205.4401) (36.426, -205.702) (36.3074, -205.8279) knots 0 0 0 1 2 2 2
  spline S119 degree 2 poles (36.3074, -205.8279) (36.1147, -206.0379) (35.643, -206.4874) (35.5022, -206.6183) knots 0 0 0 1 2 2 2
  line L90 (35.5022, -206.6183) -> (36.999, -206.6183)
  line L91 (36.999, -206.6183) -> (36.999, -206.9716)
  spline S120 degree 2 poles (39.3332, -205.9835) (39.3332, -206.2182) (39.1776, -206.6159) (39.0466, -206.7493) knots 0 0 0 1 2 2 2
  spline S121 degree 2 poles (39.0466, -206.7493) (38.9108, -206.89) (38.5699, -207.0358) (38.3649, -207.0358) knots 0 0 0 1 2 2 2
  spline S122 degree 2 poles (38.3649, -207.0358) (38.1599, -207.0358) (37.8215, -206.8975) (37.6931, -206.7591) knots 0 0 0 1 2 2 2
  spline S123 degree 2 poles (37.6931, -206.7591) (37.535, -206.5936) (37.3572, -206.0379) (37.3572, -205.6328) knots 0 0 0 1 2 2 2
  spline S124 degree 2 poles (37.3572, -205.6328) (37.3572, -205.2351) (37.5202, -204.5954) (37.6906, -204.3583) knots 0 0 0 1 2 2 2
  spline S125 degree 2 poles (37.6906, -204.3583) (37.8561, -204.1261) (38.3797, -203.8667) (38.7231, -203.8667) knots 0 0 0 1 2 2 2
  spline S126 degree 2 poles (38.7231, -203.8667) (38.8243, -203.8667) (39.0022, -203.8865) (39.0689, -203.9087) knots 0 0 0 1 2 2 2
  line L92 (39.0689, -203.9087) -> (39.0689, -204.3015)
  line L93 (39.0689, -204.3015) -> (39.0516, -204.3015)
  spline S127 degree 2 poles (39.0516, -204.3015) (38.9948, -204.2718) (38.7873, -204.22) (38.6687, -204.22) knots 0 0 0 1 2 2 2
  spline S128 degree 2 poles (38.6687, -204.22) (38.2883, -204.22) (37.8215, -204.7337) (37.7771, -205.2376) knots 0 0 0 1 2 2 2
  spline S129 degree 2 poles (37.7771, -205.2376) (37.9228, -205.1363) (38.2291, -205.0252) (38.4118, -205.0252) knots 0 0 0 1 2 2 2
  spline S130 degree 2 poles (38.4118, -205.0252) (38.5897, -205.0252) (38.8565, -205.0968) (39.0022, -205.2055) knots 0 0 0 1 2 2 2
  spline S131 degree 2 poles (39.0022, -205.2055) (39.1701, -205.3315) (39.3332, -205.7217) (39.3332, -205.9835) knots 0 0 0 1 2 2 2
  spline S132 degree 2 poles (38.9182, -206.0008) (38.9182, -205.8131) (38.8194, -205.5587) (38.7107, -205.4698) knots 0 0 0 1 2 2 2
  spline S133 degree 2 poles (38.7107, -205.4698) (38.6292, -205.4056) (38.4267, -205.3636) (38.3205, -205.3636) knots 0 0 0 1 2 2 2
  spline S134 degree 2 poles (38.3205, -205.3636) (38.1772, -205.3636) (37.908, -205.45) (37.7771, -205.5315) knots 0 0 0 1 2 2 2
  spline S135 degree 2 poles (37.7771, -205.5315) (37.7746, -205.576) (37.7696, -205.66) (37.7696, -205.7242) knots 0 0 0 1 2 2 2
  spline S136 degree 2 poles (37.7696, -205.7242) (37.7696, -206.0404) (37.8931, -206.4281) (37.987, -206.5294) knots 0 0 0 1 2 2 2
  spline S137 degree 2 poles (37.987, -206.5294) (38.0735, -206.6258) (38.2612, -206.7023) (38.3674, -206.7023) knots 0 0 0 1 2 2 2
  spline S138 degree 2 poles (38.3674, -206.7023) (38.6144, -206.7023) (38.9182, -206.3516) (38.9182, -206.0008) knots 0 0 0 1 2 2 2
  point P0 (0, 0)
  constraints: 2 other
emboss "Emboss1" sketch "Sketch14" operation cut depth 2.54 direction (-1, 0, 0)
body "Solid1"
